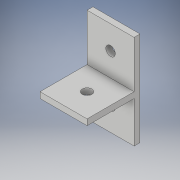
# Autodesk Inventor part: spring connector
Saved by Autodesk Inventor 2018 (Build 220112000, 112)
## iProperties
Created: 2019-01-26
Part Number: spring connector
Material: Generic
Document SubType Name: Modeling
Designer: s-2513225
Density: 1 g/cm^3
Appearance: Default
Author: s-2513225
Autodesk Inventor part; units mm, degrees
ref_plane "YZ Plane" through (0, 0, 0) normal (1, 0, 0) x (0, 1, 0)
ref_plane "XZ Plane" through (0, 0, 0) normal (0, 1, 0) x (-1, 0, 0)
sketch "Sketch1" plane through (0, 0, 0) normal (0, 0, 1) x (1, 0, 0)
  line L0 (0, 0) -> (25.4, 0)
  line L1 (25.4, 0) -> (25.4, 50.8)
  line L2 (25.4, 50.8) -> (0, 50.8)
  line L3 (0, 50.8) -> (0, 0)
  line L4 (12.7, 0) -> (12.7, 12.7) construction
  circle A0 centre (12.7, 12.7) radius 2.5797
  line L5 (12.7, 50.8) -> (12.7, 38.1) construction
  circle A1 centre (12.7, 38.1) radius 2.5797
  dimension "d0" = 25.4
  dimension "d1" = 50.8
  dimension "d13" = 12.7
  dimension "d14" = 5.1594
  dimension "d15" = 12.7
  dimension "d16" = 5.1594
  constraints: 12 end point, 2 centre point, 2 coincident, 2 midpoint, 2 parallel, 2 vertical, 1 horizontal, 1 perpendicular
  measures "d0" distance of L2.end L1.end
  measures "d1" distance of L1.end L0.end
  measures "d13" distance of L4.start L4.end
  measures "d14" diameter of A0
  measures "d15" distance of L5.start L5.end
  measures "d16" diameter of A1
ref_plane "Work Plane1" through (0, 25.4, 0) normal (0, -1, 0) x (1, 0, 0)
sketch "Sketch2" plane through (0, 25.4, 0) normal (0, -1, 0) x (1, 0, 0)
  line L0 (0, 3.175) -> (25.4, 3.175) projected
  line L1 (0, 3.175) -> (25.4, 3.175)
  line L2 (25.4, 3.175) -> (25.4, 28.575)
  line L3 (25.4, 28.575) -> (0, 28.575)
  line L4 (0, 28.575) -> (0, 3.175)
  line L5 (12.7, 28.575) -> (12.7, 15.875) construction
  circle A0 centre (12.7, 15.875) radius 2.5797
  point P0 (0, 0)
  dimension "d5" = 25.4
  dimension "d6" = 25.4
  dimension "d9" = 12.7
  dimension "d10" = 5.1594
  constraints: 10 end point, 2 parallel, 1 centre point, 1 coincident, 1 horizontal, 1 midpoint, 1 perpendicular, 1 vertical
  measures "d5" distance of L3.end L2.end
  measures "d6" distance of L2.end L1.end
  measures "d9" distance of L5.start L5.end
  measures "d10" diameter of A0
extrude "Extrusion3" add sketch "Sketch2" along normal blind 3.175
extrude "Extrusion4" add sketch "Sketch1" along normal blind 3.175
body "Solid1"
